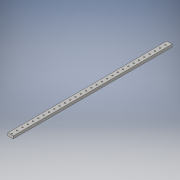
# Autodesk Inventor part: Table Pattern
Saved by Autodesk Inventor 2016 (Build 200138000, 138)
## iProperties
Created: 2015-06-03
Part Number: Table Pattern
Material: Generic
Document SubType Name: Modeling
Designer: Dennis
Density: 1 g/cm^3
Appearance: Default
Author: Dennis
Autodesk Inventor part; units mm, degrees
ref_plane "YZ Plane" through (0, 0, 0) normal (1, 0, 0) x (0, 1, 0)
ref_plane "XZ Plane" through (0, 0, 0) normal (0, 1, 0) x (-1, 0, 0)
ref_plane "XY Plane" through (0, 0, 0) normal (0, 0, 1) x (1, 0, 0)
sketch "Sketch1" plane through (0, 0, 0) normal (0, 1, 0) x (-1, 0, 0)
  line L0 (0, 0) -> (25.4, 0)
  line L1 (25.4, 0) -> (25.4, -762)
  line L2 (25.4, -762) -> (0, -762)
  line L3 (0, -762) -> (0, 0)
  circle A0 centre (12.7, -6.35) radius 3.175
  circle A1 centre (12.7, -31.75) radius 3.175
  circle A2 centre (12.7, -57.15) radius 3.175
  circle A3 centre (12.7, -82.55) radius 3.175
  circle A4 centre (12.7, -107.95) radius 3.175
  circle A5 centre (12.7, -133.35) radius 3.175
  circle A6 centre (12.7, -158.75) radius 3.175
  circle A7 centre (12.7, -184.15) radius 3.175
  circle A8 centre (12.7, -209.55) radius 3.175
  circle A9 centre (12.7, -234.95) radius 3.175
  circle A10 centre (12.7, -260.35) radius 3.175
  circle A11 centre (12.7, -285.75) radius 3.175
  circle A12 centre (12.7, -311.15) radius 3.175
  circle A13 centre (12.7, -336.55) radius 3.175
  circle A14 centre (12.7, -361.95) radius 3.175
  circle A15 centre (12.7, -387.35) radius 3.175
  circle A16 centre (12.7, -412.75) radius 3.175
  circle A17 centre (12.7, -438.15) radius 3.175
  circle A18 centre (12.7, -463.55) radius 3.175
  circle A19 centre (12.7, -488.95) radius 3.175
  circle A20 centre (12.7, -514.35) radius 3.175
  circle A21 centre (12.7, -539.75) radius 3.175
  circle A22 centre (12.7, -565.15) radius 3.175
  circle A23 centre (12.7, -590.55) radius 3.175
  circle A24 centre (12.7, -615.95) radius 3.175
  circle A25 centre (12.7, -641.35) radius 3.175
  circle A26 centre (12.7, -666.75) radius 3.175
  circle A27 centre (12.7, -692.15) radius 3.175
  circle A28 centre (12.7, -717.55) radius 3.175
  circle A29 centre (12.7, -742.95) radius 3.175
  dimension "d0" = 762
  dimension "d1" = 25.4
  dimension "d2" = 6.35
  dimension "d3" = 6.35
  dimension "d6" = 25.4
  constraints: 30 centre point, 8 end point, 2 parallel, 1 horizontal, 1 perpendicular, 1 vertical, 58 other
  measures "d0" distance of L2.end L0.start
  measures "d1" distance of L0.start L0.end
  measures "d2" diameter of A0
  measures "d3" distance from line of L0 A0.centre
  measures "d6" distance of A0.centre A1.centre
extrude "Extrusion1" add sketch "Sketch1" along normal blind 12.7
body "Solid1"
